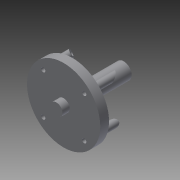
# Autodesk Inventor part: inner bayonet connector 8
Saved by Autodesk Inventor 2015 (Build 190159000, 159)
## iProperties
Created: 2014-06-10
Part Number: inner bayonet connector 8
Material: Generic
Document SubType Name: Modeling
Designer: ericd_000
Density: 1 g/cm^3
Appearance: Default
Author: ericd_000
Autodesk Inventor part; units mm, degrees
ref_plane "YZ Plane" through (0, 0, 0) normal (1, 0, 0) x (0, 1, 0)
ref_plane "XZ Plane" through (0, 0, 0) normal (0, 1, 0) x (-1, 0, 0)
ref_plane "XY Plane" through (0, 0, 0) normal (0, 0, 1) x (1, 0, 0)
sketch "Sketch1" plane through (0, 0, 0) normal (0, 1, 0) x (-1, 0, 0)
  circle A0 centre (0, 0) radius 25
  circle A1 centre (0, 0) radius 5.5
  circle A2 centre (14, 14) radius 3
  circle A3 centre (-14, 14) radius 3
  circle A4 centre (-14, -14) radius 3
  circle A5 centre (14, -14) radius 3
  line L0 (14, 14) -> (14, -14) construction
  line L1 (14, -14) -> (-14, -14) construction
  point P0 (14, 0)
  point P1 (0, -14)
  dimension "d0" = 50
  dimension "d1" = 11
  dimension "d2" = 6
  dimension "d3" = 6
  dimension "d4" = 6
  dimension "d5" = 6
  dimension "d6" = 28
  dimension "d7" = 28
  dimension "d8" = 28
  dimension "d9" = 28
  constraints: 6 centre point, 4 end point, 2 coincident, 2 midpoint, 1 horizontal, 1 horizontal alignment, 1 vertical, 1 vertical alignment
  measures "d0" diameter of A0
  measures "d1" diameter of A1
  measures "d2" diameter of A2
  measures "d3" diameter of A5
  measures "d4" diameter of A4
  measures "d5" diameter of A3
  measures "d6" distance of L0.end L0.start
  measures "d7" distance of A3.centre L0.start
  measures "d8" distance of L1.end A3.centre
  measures "d9" distance of L0.end L1.end
extrude "Extrusion2" add sketch "Sketch1" along normal blind 10 contours A1 | A2 | A3 | A4 | A5
sketch "Sketch5" plane through (0, 0, 0) normal (0, -1, 0) x (1, 0, 0)
  circle A0 centre (0, 0) radius 25
  circle A1 centre (0, 0) radius 25
  line L0 (14, 14) -> (14, -14) construction
  line L1 (14, -14) -> (-14, -14) construction
  point P0 (14, 0)
  point P1 (0, -14)
  dimension "d17" = 50
  dimension "d20" = 50
  dimension "d29" = 28
  constraints: 4 end point, 2 centre point, 2 coincident, 2 midpoint, 1 horizontal, 1 horizontal alignment, 1 vertical, 1 vertical alignment
  measures "d17" diameter of A0
  measures "d20" diameter of A1
  measures "d29" distance of L0.end L1.end
extrude "Extrusion5" add sketch "Sketch5" along normal blind 6
sketch "Sketch7" plane through (14, 10, 14) normal (0, 1, 0) x (1, 0, 0)
  circle A0 centre (0, 0) radius 2.5
  circle A1 centre (0, 0) radius 3 projected
  point P0 (-14, 14)
  dimension "d34" = 5
  constraints: 1 centre point, 1 concentric
  measures "d34" diameter of A0
extrude "Extrusion7" cut sketch "Sketch7" against normal blind 10
sketch "Sketch8" plane through (14, 10, -14) normal (0, 1, 0) x (1, 0, 0)
  circle A0 centre (0, 0) radius 2.5
  circle A1 centre (0, 0) radius 3 projected
  point P0 (-14, -14)
  dimension "d37" = 5
  constraints: 1 centre point, 1 concentric
  measures "d37" diameter of A0
extrude "Extrusion8" cut sketch "Sketch8" against normal blind 10
sketch "Sketch9" plane through (-14, 10, -14) normal (0, 1, 0) x (1, 0, 0)
  circle A0 centre (0, 0) radius 2.5
  circle A1 centre (0, 0) radius 3 projected
  point P0 (14, -14)
  dimension "d40" = 5
  constraints: 1 centre point, 1 concentric
  measures "d40" diameter of A0
extrude "Extrusion9" cut sketch "Sketch9" against normal blind 10
sketch "Sketch10" plane through (-14, 10, 14) normal (0, 1, 0) x (1, 0, 0)
  circle A0 centre (0, 0) radius 2.5
  circle A1 centre (0, 0) radius 3 projected
  point P0 (14, 14)
  dimension "d43" = 5
  constraints: 1 centre point, 1 concentric
  measures "d43" diameter of A0
extrude "Extrusion10" cut sketch "Sketch10" against normal blind 10
sketch "Sketch26" plane through (0, 10, 0) normal (0, 1, 0) x (1, 0, 0)
  circle A0 centre (14, 14) radius 2.5 projected
  circle A1 centre (14, 14) radius 2.5
  circle A2 centre (14, -14) radius 2.5
  circle A3 centre (14, -14) radius 2.5 projected
  line L0 (11.5099, -14.2224) -> (13.9901, -11.5)
  line L1 (13.9901, -11.5) -> (16.4901, -13.7776)
  line L2 (16.4901, -13.7776) -> (14.0099, -16.5)
  line L3 (14.0099, -16.5) -> (11.5099, -14.2224)
  line L4 (13.9901, 11.5) -> (11.5099, 13.7777)
  line L5 (11.5099, 13.7777) -> (14.0099, 16.5)
  line L6 (14.0099, 16.5) -> (16.4901, 14.2223)
  line L7 (16.4901, 14.2223) -> (13.9901, 11.5)
  circle A4 centre (0, 0) radius 5.5 projected
  circle A5 centre (0, 0) radius 19.799
  circle A6 centre (-14, 14) radius 2.5
  circle A7 centre (-14, 14) radius 2.5 projected
  line L8 (-13.7777, 11.5099) -> (-16.5, 14.0099)
  line L9 (-16.5, 14.0099) -> (-14.2223, 16.4901)
  line L10 (-14.2223, 16.4901) -> (-11.5, 13.9901)
  line L11 (-11.5, 13.9901) -> (-13.7777, 11.5099)
  circle A8 centre (-14, -14) radius 2.5
  circle A9 centre (-14, -14) radius 2.5 projected
  line L12 (-16.5, -14.0099) -> (-14.2224, -11.5099)
  line L13 (-14.2224, -11.5099) -> (-11.5, -13.9901)
  line L14 (-11.5, -13.9901) -> (-13.7776, -16.4901)
  line L15 (-13.7776, -16.4901) -> (-16.5, -14.0099)
  point P0 (15.2401, -12.6388)
  point P1 (12.7599, 15.1389)
  point P2 (-15.1389, 12.7599)
  point P3 (-12.6388, -15.2401)
  dimension "d100" = 5
  dimension "d101" = 90
  dimension "d104" = 90
  dimension "d106" = 90
  dimension "d112" = 2.5
  dimension "d113" = 2.5
  dimension "d114" = 2.4802
  dimension "d115" = 2.4802
  dimension "d116" = 5
  dimension "d117" = 90
  dimension "d118" = 2.5
  dimension "d119" = 5
  dimension "d120" = 90
  dimension "d121" = 90
  dimension "d122" = 2.5
  constraints: 32 end point, 22 point on circle, 6 parallel, 5 centre point, 4 midpoint, 3 concentric, 2 coincident, 2 perpendicular
  measures "d100" diameter of A2
  measures "d101" angle of L0 L1
  measures "d104" angle of L7 L4
  measures "d106" angle of L4 L5
  measures "d112" horizontal distance of L0.end L1.end
  measures "d113" horizontal distance of L4.end L5.end
  measures "d114" horizontal distance of L0.start L0.end
  measures "d115" horizontal distance of L4.start L4.end
  measures "d116" diameter of A6
  measures "d117" angle of L9 L8
  measures "d118" vertical distance of L8.start L8.end
  measures "d119" diameter of A8
  measures "d120" angle of L12 L15
  measures "d121" angle of L14 L15
  measures "d122" vertical distance of L13.end L14.end
extrude "Extrusion22" add sketch "Sketch26" along normal blind 5 contours L7 A5 L5 L6 | L7 L4 L5 A5 | L2 L3 A5 L1 | L1 A5 L3 L0 | L10 L11 L8 A5 | A5 L8 L9 L10 | L14 L15 L12 A5 | A5 L12 L13 L14
chamfer "Chamfer3" distance 3.35 angle 45 4 edges at (-12.6388, 15, 15.2401) (-15.1389, 15, -12.7599) (15.2401, 15, 12.6388) (12.7599, 15, -15.1389)
sketch "Sketch31" plane through (0, 10, 0) normal (0, 1, 0) x (1, 0, 0)
  line L0 (14.0099, -16.5) -> (16.4901, -13.7776)
  line L1 (14.0099, -16.5) -> (11.5099, -14.2224) projected
  arc A0 (14.0099, -16.5) -> (16.4901, -13.7776) centre (14, -14) ccw
  line L2 (11.5099, -14.2224) -> (13.9901, -11.5)
  line L3 (13.9901, -11.5) -> (16.4901, -13.7776) projected
  arc A1 (13.9901, -11.5) -> (11.5099, -14.2224) centre (14, -14) ccw
  point P0 (0, 0)
  constraints: 4 end point, 4 point on circle, 2 centre point, 2 perpendicular
extrude "Extrusion26" add sketch "Sketch31" along normal up to surface contours L0 A0 | A1 L2 surface through (14.737, 13.325, 14.4464) normal (0.4762083, 0.7071068, -0.5227099)
sketch "Sketch32" plane through (0, 10, 0) normal (0, 1, 0) x (1, 0, 0)
  line L0 (16.4901, 14.2223) -> (14.0099, 16.5)
  arc A0 (16.4901, 14.2223) -> (14.0099, 16.5) centre (14, 14) ccw
  arc A1 (16.4901, 14.2223) -> (14.0099, 16.5) centre (14, 14) ccw projected
  arc A2 (11.5099, 13.7777) -> (13.9901, 11.5) centre (14, 14) ccw
  line L1 (11.5099, 13.7777) -> (13.9901, 11.5)
  line L2 (13.9901, 11.5) -> (11.5099, 13.7777) projected
  point P0 (0, 0)
  constraints: 4 end point, 4 point on circle, 2 centre point, 1 collinear, 1 concentric
extrude "Extrusion27" add sketch "Sketch32" along normal up to surface surface through (13.9936, 13.325, -14.0059) normal (-0.5208077, 0.7071068, -0.4782879)
sketch "Sketch33" plane through (0, 10, 0) normal (0, 1, 0) x (1, 0, 0)
  line L0 (13.9901, 11.5) -> (16.4901, 14.2223)
  line L1 (16.4901, 14.2223) -> (13.9901, 11.5) projected
  arc A0 (13.9901, 11.5) -> (16.4901, 14.2223) centre (14, 14) ccw
  point P0 (0, 0)
  constraints: 2 end point, 2 point on circle, 1 centre point, 1 collinear
extrude "Extrusion28" add sketch "Sketch33" along normal blind 5
sketch "Sketch34" plane through (0, 10, 0) normal (0, 1, 0) x (1, 0, 0)
  line L0 (11.5099, -14.2224) -> (14.0099, -16.5)
  line L1 (14.0099, -16.5) -> (11.5099, -14.2224) projected
  arc A0 (11.5099, -14.2224) -> (14.0099, -16.5) centre (14, -14) ccw
  point P0 (0, 0)
  constraints: 2 end point, 2 point on circle, 1 centre point, 1 collinear
extrude "Extrusion29" add sketch "Sketch34" along normal blind 5
sketch "Sketch35" plane through (14.0099, 15, 16.5) normal (-0.7392234, 0, -0.6734602) x (-0.6734602, 0, 0.7392234)
  line L0 (0, 0) -> (-0.3327, 0)
  line L1 (-0.3327, 0) -> (0, 0.3327)
  line L2 (-3.6827, -3.35) -> (0, 0.3327) projected
  line L3 (0, 0.3327) -> (0, 0)
  point P0 (-2.7621, -15)
  constraints: 6 end point, 1 collinear, 1 horizontal, 1 perpendicular
extrude "Extrusion30" cut sketch "Sketch35" along normal mid plane 10
sketch "Sketch36" plane through (0, 10, 0) normal (0, 1, 0) x (1, 0, 0)
  line L0 (-16.5, -14.0099) -> (-13.7776, -16.4901)
  line L1 (-11.5, -13.9901) -> (-14.2224, -11.5099)
  line L2 (-14.2224, -11.5099) -> (-11.5, -13.9901) projected
  arc A0 (-16.5, -14.0099) -> (-13.7776, -16.4901) centre (-14, -14) ccw
  arc A1 (-11.5, -13.9901) -> (-14.2224, -11.5099) centre (-14, -14) ccw
  point P0 (0, 0)
  constraints: 4 end point, 4 point on circle, 2 centre point, 1 collinear
extrude "Extrusion31" add sketch "Sketch36" along normal up to surface surface through (-13.877, 13.325, 14.112) normal (0.5227099, 0.7071068, 0.4762083)
sketch "Sketch37" plane through (0, 10, 0) normal (0, 1, 0) x (1, 0, 0)
  line L0 (-14.2224, -11.5099) -> (-16.5, -14.0099)
  line L1 (-16.5, -14.0099) -> (-14.2224, -11.5099) projected
  arc A0 (-14.2224, -11.5099) -> (-16.5, -14.0099) centre (-14, -14) ccw
  point P0 (0, 0)
  constraints: 2 end point, 2 point on circle, 1 centre point, 1 collinear
extrude "Extrusion32" add sketch "Sketch37" along normal blind 5
sketch "Sketch38" plane through (-16.5, 15, 14.0099) normal (0.6734602, 0, -0.7392234) x (-0.7392234, 0, -0.6734602)
  line L0 (-0.3327, 0) -> (0, 0)
  line L1 (0, 0) -> (0, 0.3327)
  line L2 (0, 0) -> (0, 0.3327) projected
  line L3 (0, 0.3327) -> (-0.3327, 0)
  point P0 (-2.7621, -15)
  constraints: 6 end point, 1 collinear, 1 horizontal
extrude "Extrusion33" cut sketch "Sketch38" along normal mid plane 10
sketch "Sketch39" plane through (0, 10, 0) normal (0, 1, 0) x (1, 0, 0)
  point P0 (0, 0)
sketch "Sketch40" plane through (0, 10, 0) normal (0, 1, 0) x (1, 0, 0)
  line L0 (-14.2223, 16.4901) -> (-16.5, 14.0099)
  arc A0 (-14.2223, 16.4901) -> (-16.5, 14.0099) centre (-14, 14) ccw
  arc A1 (-13.7777, 11.5099) -> (-11.5, 13.9901) centre (-14, 14) ccw
  line L1 (-11.5, 13.9901) -> (-13.7777, 11.5099)
  line L2 (-11.5, 13.9901) -> (-13.7777, 11.5099) projected
  point P0 (0, 0)
  constraints: 4 end point, 4 point on circle, 2 centre point, 1 collinear
extrude "Extrusion34" add sketch "Sketch40" along normal up to surface surface through (-14.0059, 13.325, -13.9936) normal (-0.4782879, 0.7071068, 0.5208077)
sketch "Sketch41" plane through (0, 10, 0) normal (0, 1, 0) x (1, 0, 0)
  line L0 (-14.2223, 16.4901) -> (-11.5, 13.9901)
  line L1 (-14.2223, 16.4901) -> (-11.5, 13.9901) projected
  arc A0 (-11.5, 13.9901) -> (-14.2223, 16.4901) centre (-14, 14) ccw
  point P0 (0, 0)
  constraints: 2 end point, 2 point on circle, 1 centre point, 1 collinear
extrude "Extrusion35" add sketch "Sketch41" along normal blind 5
sketch "Sketch42" plane through (0, 10, 0) normal (0, 1, 0) x (1, 0, 0)
  line L0 (-16.5, 14.0099) -> (-13.7777, 11.5099)
  arc A0 (-16.5, 14.0099) -> (-13.7777, 11.5099) centre (-14, 14) ccw
  point P0 (0, 0)
  constraints: 2 end point, 2 point on circle, 1 centre point
extrude "Extrusion36" add sketch "Sketch42" along normal up to surface (1.65 mm away)
sketch "Sketch43" plane through (-14, 11.65, -14) normal (0, 1, 0) x (0.7365333, 0, 0.6764013)
  line L0 (-1.848, -1.6837) -> (1.848, -1.6837)
  line L1 (-1.848, -1.6837) -> (1.848, -1.6837) projected
  arc A0 (-1.848, -1.6837) -> (1.848, -1.6837) centre (0, 0) ccw
  arc A1 (-1.848, -1.6837) -> (1.848, -1.6837) centre (0, 0) ccw projected
  point P0 (19.7811, -0.8418)
  constraints: 2 end point, 2 point on circle, 1 centre point, 1 collinear, 1 concentric
extrude "Extrusion37" cut sketch "Sketch43" along normal up to surface surface through (-14.0059, 13.325, -13.9936) normal (-0.4782879, 0.7071068, 0.5208077)
sketch "Sketch44" plane through (0, 10, 0) normal (0, 1, 0) x (1, 0, 0)
  line L0 (14.0099, 16.5) -> (11.5099, 13.7777)
  arc A0 (14.0099, 16.5) -> (11.5099, 13.7777) centre (14, 14) ccw
  arc A1 (14.0099, 16.5) -> (11.5099, 13.7777) centre (14, 14) ccw projected
  point P0 (0, 0)
  constraints: 2 end point, 2 point on circle, 1 centre point, 1 concentric
extrude "Extrusion38" add sketch "Sketch44" along normal up to surface (1.65 mm away)
sketch "Sketch45" plane through (14, 11.65, -14) normal (0, 1, 0) x (0.7365333, 0, 0.6764013)
  line L0 (-1.6837, 1.848) -> (-1.6837, -1.848)
  arc A0 (-1.6837, 1.848) -> (-1.6837, -1.848) centre (0, 0) ccw
  point P0 (-0.8418, -19.7811)
  constraints: 2 end point, 2 point on circle, 1 centre point, 1 vertical
extrude "Extrusion39" cut sketch "Sketch45" along normal up to surface surface through (13.9936, 13.325, -14.0059) normal (-0.5208077, 0.7071068, -0.4782879)
sketch "Sketch46" plane through (0, 10, 0) normal (0, 1, 0) x (1, 0, 0)
  line L0 (16.4901, -13.7776) -> (14, -11.509)
  line L1 (13.9901, -11.5) -> (16.4901, -13.7776) projected
  arc A0 (16.4901, -13.7776) -> (13.9901, -11.5) centre (14, -14) ccw
  point P0 (0, 0)
  constraints: 2 end point, 2 point on circle, 1 centre point, 1 collinear
extrude "Extrusion40" add sketch "Sketch46" along normal up to surface (1.65 mm away)
sketch "Sketch47" plane through (14, 11.65, 14) normal (0, 1, 0) x (0.7392234, 0, 0.6734602)
  line L0 (-1.691, 1.8414) -> (1.691, 1.8414)
  line L1 (1.691, 1.8414) -> (-1.691, 1.8414) projected
  arc A0 (1.691, 1.8414) -> (-1.691, 1.8414) centre (0, 0) ccw
  arc A1 (-1.691, 1.8414) -> (-1.9935, -1.5086) centre (0, 0) ccw projected
  point P0 (-19.7776, 0.9207)
  constraints: 2 end point, 2 point on circle, 1 centre point, 1 collinear, 1 concentric
extrude "Extrusion41" cut sketch "Sketch47" along normal up to surface surface through (14.737, 13.325, 14.4464) normal (0.4762083, 0.7071068, -0.5227099)
sketch "Sketch48" plane through (0, 10, 0) normal (0, 1, 0) x (1, 0, 0)
  line L0 (-11.5, -13.9901) -> (-13.7776, -16.4901)
  line L1 (-11.5, -13.9901) -> (-13.7776, -16.4901) projected
  arc A0 (-13.7776, -16.4901) -> (-11.5, -13.9901) centre (-14, -14) ccw
  point P0 (0, 0)
  constraints: 2 end point, 2 point on circle, 1 centre point, 1 collinear
extrude "Extrusion42" add sketch "Sketch48" along normal up to surface surface through (-13.877, 13.325, 14.112) normal (0.5227099, 0.7071068, 0.4762083)
sketch "Sketch49" plane through (0, 15, 0) normal (0, 1, 0) x (1, 0, 0)
  point P0 (0, 0)
sketch "Sketch50" plane through (0, 15, 0) normal (0, 1, 0) x (1, 0, 0)
  line L0 (11.5104, -13.7727) -> (14.4576, -16.4578)
  line L1 (11.5104, -13.7727) -> (14.4576, -16.4578) projected
  arc A0 (11.5104, -13.7727) -> (14.4576, -16.4578) centre (14, -14) ccw
  point P0 (0, 0)
  constraints: 2 end point, 2 point on circle, 1 centre point, 1 collinear
extrude "Extrusion43" add sketch "Sketch50" against normal up to surface surface through (14.737, 13.325, 14.4464) normal (0.4762083, 0.7071068, -0.5227099)
sketch "Sketch51" plane through (0, 15, 0) normal (0, 1, 0) x (1, 0, 0)
  line L0 (-16.4578, -14.4576) -> (-13.7727, -11.5104)
  line L1 (-13.7727, -11.5104) -> (-16.4578, -14.4576) projected
  arc A0 (-13.7727, -11.5104) -> (-16.4578, -14.4576) centre (-14, -14) ccw
  point P0 (0, 0)
  constraints: 2 end point, 2 point on circle, 1 centre point, 1 collinear
extrude "Extrusion44" add sketch "Sketch51" against normal up to surface surface through (-13.877, 13.325, 14.112) normal (0.5227099, 0.7071068, 0.4762083)
sketch "Sketch52" plane through (0, 15, 0) normal (0, 1, 0) x (1, 0, 0)
  line L0 (-14.234, 16.4773) -> (-11.5118, 13.9773)
  line L1 (-11.5118, 13.9773) -> (-14.234, 16.4773) projected
  arc A0 (-11.5, 13.9901) -> (-14.2223, 16.4901) centre (-14, 14) ccw
  arc A1 (-11.5, 13.9901) -> (-14.2223, 16.4901) centre (-14, 14) ccw projected
  line L2 (16.4773, 14.234) -> (13.9773, 11.5118)
  line L3 (13.9773, 11.5118) -> (16.4773, 14.234) projected
  arc A2 (13.9773, 11.5118) -> (16.4773, 14.234) centre (14.0263, 13.9759) ccw
  point P0 (0, 0)
  constraints: 4 end point, 4 point on circle, 2 centre point, 2 collinear, 1 concentric
extrude "Extrusion46" add sketch "Sketch52" against normal up to surface surface through (13.9936, 13.325, -14.0059) normal (-0.5208077, 0.7071068, -0.4782879)
sketch "Sketch53" plane through (0, 15, 0) normal (0, 1, 0) x (1, 0, 0)
  line L0 (-11.5, 13.9901) -> (-14.2223, 16.4901)
  line L1 (-11.5118, 13.9773) -> (-14.234, 16.4773) projected
  arc A0 (-11.5118, 13.9773) -> (-14.234, 16.4773) centre (-13.9757, 14.0265) ccw
  point P0 (0, 0)
  constraints: 2 end point, 2 point on circle, 1 centre point, 1 parallel
extrude "Extrusion47" add sketch "Sketch53" against normal up to surface surface through (-14.0059, 13.325, -13.9936) normal (-0.4782879, 0.7071068, 0.5208077)
sketch "Sketch54" plane through (0, 10, 0) normal (0, 1, 0) x (1, 0, 0)
  circle A0 centre (0, 0) radius 5.5
  constraints: 1 centre point, 1 coincident
extrude "Extrusion48" add sketch "Sketch54" along normal blind 25
sketch "Sketch55" plane through (0, -6, 0) normal (0, -1, 0) x (1, 0, 0)
  point P0 (0, 0)
sketch "Sketch56" plane through (0, 0, 0) normal (0, 1, 0) x (1, 0, 0)
  point P0 (0, 0)
sketch "Sketch59" plane through (0, 0, 0) normal (0, 1, 0) x (1, 0, 0)
  circle A0 centre (14, -14) radius 1.5
  circle A1 centre (14, -14) radius 2.5 projected
  point P0 (0, 0)
  dimension "d186" = 1
  constraints: 1 centre point, 1 concentric
  measures "d186" radial gap between concentric circles of A1 A0
extrude "Extrusion49" cut sketch "Sketch59" along normal through all both and the other way through all contours A0
pattern_circular "Circular Pattern1" count 4 over 360 about axis through (0, 0, 0) along (0, 1, 0) of "Extrusion49"
sketch "Sketch60" plane through (0, -6, 0) normal (0, -1, 0) x (1, 0, 0)
  circle A0 centre (0, 0) radius 4.2
  dimension "d192" = 8.4
  constraints: 1 centre point, 1 coincident
  measures "d192" diameter of A0
extrude "Extrusion50" add sketch "Sketch60" along normal blind 5
body "Solid2"
